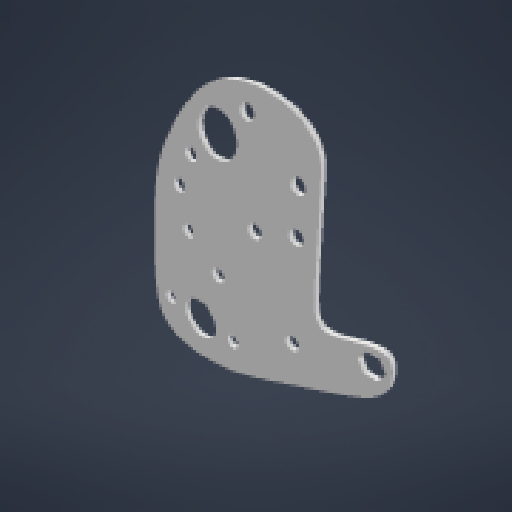
# Autodesk Inventor part: third-stage
Saved by Autodesk Inventor 2023 (Build 270158000, 158)
## iProperties
Created: 2023-03-29
Part Number: third-stage
Material: Generic
Document SubType Name: Modeling
Designer: Liam
Density: 1 g/cm^3
Appearance: Default
Author: Liam
Autodesk Inventor part; units mm, degrees
ref_plane "YZ Plane" through (0, 0, 0) normal (1, 0, 0) x (0, 1, 0)
ref_plane "XZ Plane" through (0, 0, 0) normal (0, 1, 0) x (-1, 0, 0)
ref_plane "XY Plane" through (0, 0, 0) normal (0, 0, 1) x (1, 0, 0)
sketch "Sketch1" plane through (0, 0, 0) normal (0, 0, 1) x (1, 0, 0)
  circle A0 centre (-45.6184, 44.45) radius 2.0955
  circle A1 centre (-45.6184, 57.15) radius 2.0955
  circle A2 centre (-79.3648, 1.8096) radius 6.35
  circle A3 centre (-58.2829, 40.2547) radius 2.0955
  circle A4 centre (-84.7892, 41.664) radius 2.0955
  circle A5 centre (-66.6703, 1.4359) radius 2.0955
  circle A6 centre (-92.0593, 2.1834) radius 2.0955
  circle A7 centre (-71.4316, 20.7646) radius 2.0955
  circle A8 centre (-82.2396, 29.27) radius 2.0955
  circle A9 centre (-69.9964, 60.5103) radius 6.35
  circle A10 centre (-60.4479, 68.8837) radius 2.0955
  circle A11 centre (-79.545, 52.1369) radius 2.0955
  line L0 (-26.356, 22.0475) -> (-24.4745, 18.8943)
  line L1 (-24.4745, 18.8943) -> (-20.8087, 18.9471)
  line L2 (-20.8087, 18.9471) -> (-19.0215, 22.1481)
  line L3 (-19.0215, 22.1481) -> (-20.903, 25.3013)
  line L4 (-20.903, 25.3013) -> (-24.5688, 25.2486)
  line L5 (-24.5688, 25.2486) -> (-26.356, 22.0475)
  line L6 (-39.6875, 62.484) -> (-39.6875, 39.116)
  line L7 (-39.6875, 62.484) -> (-39.6875, 72.0287) construction
  line L8 (-39.6875, 72.0287) -> (-60.4479, 79.1818) construction
  line L9 (-60.4479, 79.1818) -> (-76.3464, 72.0287) construction
  line L10 (-76.3464, 72.0287) -> (-86.8847, 55.842) construction
  line L11 (-86.8847, 55.842) -> (-95.25, 43.7595) construction
  line L12 (-95.25, 43.7595) -> (-100.0125, 0.0879) construction
  line L13 (-100.0125, 0.0879) -> (-96.8375, -11.1125) construction
  line L14 (-96.8375, -11.1125) -> (-82.2396, -13.4359) construction
  line L15 (-82.2396, -13.4359) -> (-62.5434, -9.525) construction
  line L16 (-62.5434, -9.525) -> (-39.6875, 4.2789) construction
  line L17 (-39.6875, 4.2789) -> (-20.8087, 11.8111) construction
  line L18 (-20.8087, 11.8111) -> (-17.1458, 19.0047) construction
  line L19 (-17.1458, 19.0047) -> (-17.1458, 25.2486) construction
  line L20 (-17.1458, 25.2486) -> (-20.8087, 39.116) construction
  line L21 (-20.8087, 39.116) -> (-37.9665, 20.5476) construction
  line L22 (-37.9665, 20.5476) -> (-39.6875, 38.1592) construction
  line L23 (-39.6875, 38.1592) -> (-39.6875, 39.116) construction
  spline S0 degree 4 poles (-39.6875, 62.484) (-39.6875, 72.0287) (-60.4479, 79.1818) (-76.3464, 72.0287) (-86.8847, 55.842) (-95.25, 43.7595) (-100.0125, 0.0879) (-96.8375, -11.1125) (-82.2396, -13.4359) (-62.5434, -9.525) (-39.6875, 4.2789) (-20.8087, 11.8111) (-17.1458, 19.0047) (-17.1458, 25.2486) (-20.8087, 39.116) (-37.9665, 20.5476) (-39.6875, 38.1592) (-39.6875, 39.116) knots 1 1 1 1 1 2 3 4 5 6 7 8 9 10 11 12 13 14 15 15 15 15 15
  circle A12 centre (-45.6184, 14.099) radius 2.0955
  point P0 (0, 0)
  point P1 (-79.3931, 52.0233)
  point P2 (-60.4186, 72.0287)
  point P3 (-81.0906, 53.8995)
  dimension "d23" = 4.191
  dimension "d24" = 4.191
  dimension "d60" = 4.191
  dimension "d61" = 4.191
  dimension "d62" = 12.7
  dimension "d63" = 4.191
  dimension "d64" = 4.191
  dimension "d65" = 12.7
  dimension "d68" = 4.191
  dimension "d69" = 4.191
  dimension "d70" = 12.7
  dimension "d71" = 4.191
  dimension "d72" = 4.191
  dimension "d73" = 4.191
  constraints: 14 end point, 13 centre point, 3 parallel, 2 collinear, 1 vertical, 18 other
  measures "d23" diameter of A0
  measures "d24" diameter of A1
  measures "d60" diameter of A3
  measures "d61" diameter of A4
  measures "d62" diameter of A2
  measures "d63" diameter of A5
  measures "d64" diameter of A6
  measures "d65" distance of A2.centre A6.centre
  measures "d68" diameter of A7
  measures "d69" diameter of A8
  measures "d70" diameter of A9
  measures "d71" diameter of A10
  measures "d72" diameter of A11
  measures "d73" diameter of A12
extrude "Extrusion5" add sketch "Sketch1" along normal blind 1.524
body "Solid5"
